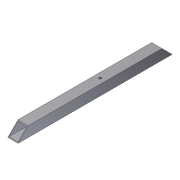
# Autodesk Inventor part: Frame_RearLowerAngleSupport
Saved by Autodesk Inventor 2012 (Build 160160000, 160)
## iProperties
Created: 2012-01-09
Part Number: Frame_RearLowerAngleSupport
Material: Default
Document SubType Name: Modeling
Designer: JesseK
Density: 1 g/cm^3
Mass: 53.7701 g
Surface Area: 681.695 cm^2
Volume: 53.7701 cm^3
Author: JesseK
Autodesk Inventor part; units mm, degrees
ref_plane "YZ Plane" through (0, 0, 0) normal (1, 0, 0) x (0, 1, 0)
ref_plane "XZ Plane" through (0, 0, 0) normal (0, 1, 0) x (-1, 0, 0)
ref_plane "XY Plane" through (0, 0, 0) normal (0, 0, 1) x (1, 0, 0)
sketch "Sketch1" plane through (0, 0, 0) normal (0, 0, 1) x (1, 0, 0)
  line L0 (0, 0) -> (25.4, 0)
  line L1 (25.4, 0) -> (25.4, 25.4)
  line L2 (25.4, 25.4) -> (0, 25.4)
  line L3 (0, 25.4) -> (0, 0)
  dimension "d0" = 25.4
  dimension "d1" = 25.4
  constraints: 8 end point, 2 parallel, 1 horizontal, 1 perpendicular
  measures "d0" distance of L1.end L2.end
  measures "d1" distance of L0.end L1.end
extrude "Extrusion1" add sketch "Sketch1" along normal blind 381
shell "Shell1" thickness 1.5875 removed faces 2 at (16.9333, 16.9333, 0) at (16.9333, 16.9333, 381)
sketch "Sketch2" plane through (25.4, 0, 0) normal (1, 0, 0) x (0, 0, -1)
  line L0 (-381, 25.4) -> (-381, 0) projected
  line L1 (0, 0) -> (0, 25.4) projected
  line L2 (0, 25.4) -> (-381, 25.4) projected
  line L3 (-381, 0) -> (-355.6, 25.4)
  line L4 (-381, 25.4) -> (-381, 0)
  line L5 (-381, 25.4) -> (-355.6, 25.4)
  line L6 (0, 25.4) -> (-25.4, 25.4)
  line L7 (0, 0) -> (-25.4, 25.4)
  line L8 (0, 0) -> (0, 25.4)
  dimension "d6" = 45
  dimension "d7" = 45
  constraints: 12 end point, 2 perpendicular, 2 point on line, 1 collinear
  measures "d6" angle of L3 L0
  measures "d7" angle of L1 L7
extrude "Extrusion2" cut sketch "Sketch2" against normal through all
sketch "Sketch3" plane through (0, 25.4, 355.6) normal (0, 1, 0) x (1, 0, 0)
  line L0 (25.4, 330.2) -> (25.4, 0) projected
  line L1 (25.4, 330.2) -> (0, 330.2) projected
  circle A0 centre (12.7, 190.5) radius 3.175
  point P0 (0, 355.6)
  dimension "d10" = 6.35
  dimension "d11" = 12.7
  dimension "d12" = 139.7
  constraints: 1 centre point
  measures "d10" diameter of A0
  measures "d11" distance from line of L0 A0.centre
  measures "d12" distance from line of L1 A0.centre
extrude "Extrusion3" cut sketch "Sketch3" against normal through all
body "Solid1"
